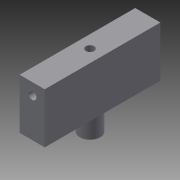
# Autodesk Inventor part: UpperTorso_v2
Saved by Autodesk Inventor 2013 (Build 170138000, 138)
## iProperties
Created: 2012-11-28
Part Number: UpperTorso_v2
Material: Generic
Document SubType Name: Modeling
Designer: Joe
Density: 1 g/cm^3
Author: Joe
Autodesk Inventor part; units mm, degrees
ref_plane "YZ Plane" through (0, 0, 0) normal (1, 0, 0) x (0, 1, 0)
ref_plane "XZ Plane" through (0, 0, 0) normal (0, 1, 0) x (-1, 0, 0)
ref_plane "XY Plane" through (0, 0, 0) normal (0, 0, 1) x (1, 0, 0)
sketch "Sketch1" plane through (0, 0, 0) normal (0, 0, 1) x (1, 0, 0)
  line L0 (0, 27) -> (138, 27)
  line L1 (138, 27) -> (138, 0)
  line L2 (138, 0) -> (138, -27)
  line L3 (138, -27) -> (27, -93) construction
  line L4 (27, -93) -> (0, -93)
  line L5 (0, -93) -> (0, 27) construction
  line L6 (0, 0) -> (138, 0) construction
  line L7 (0, 27) -> (-138, 27)
  line L8 (-138, 27) -> (-138, 0)
  line L9 (-138, 0) -> (-138, -27)
  line L10 (-138, -27) -> (-27, -93) construction
  line L11 (-27, -93) -> (0, -93)
  line L12 (27, -93) -> (138, -93)
  line L13 (138, -93) -> (138, -27)
  line L14 (-27, -93) -> (-138, -93)
  line L15 (-138, -93) -> (-138, -27)
  dimension "d0" = 138
  dimension "d2" = 27
  dimension "d3" = 54
  dimension "d4" = 27
  dimension "d5" = 120
  constraints: 32 end point, 5 symmetric about line, 3 perpendicular, 2 collinear, 2 horizontal, 1 parallel, 1 point on line
  measures "d0" distance of L0.start L0.end
  measures "d2" distance of L0.end L1.end
  measures "d3" distance of L2.end L0.end
  measures "d4" distance of L3.end L4.end
  measures "d5" distance between parallel lines of L4 L0
extrude "Extrusion1" add sketch "Sketch1" along normal mid plane 60
sketch "Sketch2" plane through (-27, -93, 30) normal (0, -1, 0) x (1, 0, 0)
  circle A0 centre (27, -30) radius 24.5
  dimension "d20" = 49
  constraints: 1 centre point, 1 coincident
  measures "d20" diameter of A0
extrude "Extrusion2" add sketch "Sketch2" along normal blind 51
sketch "Sketch3" plane through (-138, 27, 30) normal (0, 1, 0) x (1, 0, 0)
  circle A0 centre (138, 30) radius 10
  dimension "d12" = 20
  constraints: 1 centre point, 1 coincident
  measures "d12" diameter of A0
extrude "Extrusion3" cut sketch "Sketch3" against normal through all
sketch "Sketch4" plane through (138, -27, 30) normal (1, 0, 0) x (0, 0, -1)
  circle A0 centre (30, 27) radius 10
  dimension "d16" = 20
  constraints: 1 centre point, 1 coincident
  measures "d16" diameter of A0
extrude "Extrusion4" cut sketch "Sketch4" against normal through all
move or copy body "Move Body1" bodies to move or copy 1 copy no rotation origin (0, 0, 0) rotation axis (1, 0, 0) rotation angle 90
move or copy body "Move Body2" bodies to move or copy 1 copy no rotation origin (0, 0, 0) rotation axis (0, 0, 1) rotation angle 90
move or copy body "Move Body4" bodies to move or copy 1 copy no translate (0, 0, 144)
body "Solid1"
